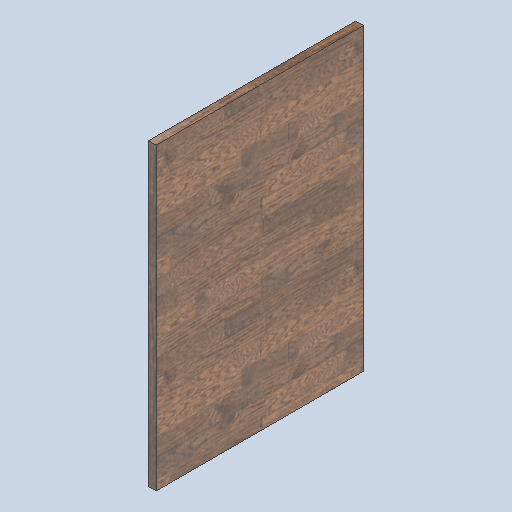
# Autodesk Inventor part: Side Panel
Saved by Autodesk Inventor 2022 (Build 260153000, 153)
## iProperties
Created: 2021-10-04
Part Number: Side Panel
Material: Generic
Document SubType Name: Modeling
Designer: Admin
Density: 1 g/cm^3
Appearance: White Ash - Java
Author: Admin
Autodesk Inventor part; units mm, degrees
ref_plane "YZ Plane" through (0, 0, 0) normal (1, 0, 0) x (0, 1, 0)
ref_plane "XZ Plane" through (0, 0, 0) normal (0, 1, 0) x (-1, 0, 0)
ref_plane "XY Plane" through (0, 0, 0) normal (0, 0, 1) x (1, 0, 0)
derived "Dresser SKELETON.ipt"
sketch "Right Panel Sketch" plane through (596.9, 0, 0) normal (1, 0, 0) x (0, 1, 0)
  line L0 (1143, -342.9) -> (152.4, -342.9)
  line L1 (1143, 342.9) -> (152.4, 342.9)
  line L2 (1143, 342.9) -> (1143, -342.9)
  line L3 (152.4, -342.9) -> (152.4, 342.9)
  point P0 (0, 0)
extrude "Extrusion1" add sketch "Right Panel Sketch" along normal blind 25.4
equation "\"d1\" = panelThickness"
equation "\"panelThickness\" = 25.4"
body "Solid1"
